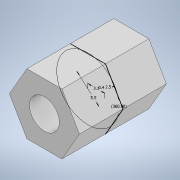
# Autodesk Inventor part: Acople_Motor_
Saved by Autodesk Inventor 2022 (Build 260153000, 153)
## iProperties
Created: 2022-03-05
Part Number: Acople_Motor_
Material: Generic
Document SubType Name: Modeling
Designer: katha
Density: 1 g/cm^3
Appearance: Default
Author: katha
Autodesk Inventor part; units mm, degrees
ref_plane "YZ Plane" through (0, 0, 0) normal (1, 0, 0) x (0, 1, 0)
ref_plane "XZ Plane" through (0, 0, 0) normal (0, 1, 0) x (-1, 0, 0)
ref_plane "XY Plane" through (0, 0, 0) normal (0, 0, 1) x (1, 0, 0)
sketch "Sketch1" plane through (0, 0, 0) normal (0, 0, 1) x (1, 0, 0)
  circle A0 centre (0, 0) radius 2.75
  line L0 (0, 0) -> (3.1, 0) construction
  line L1 (0, 0) -> (1.55, 2.6847) construction
  line L2 (0, 0) -> (-1.55, 2.6847) construction
  line L3 (0, 0) -> (-3.1, 0) construction
  line L4 (0, 0) -> (-1.55, -2.6847) construction
  line L5 (0, 0) -> (1.55, -2.6847) construction
  line L6 (-1.55, 2.6847) -> (1.55, 2.6847) construction
  line L7 (1.55, 2.6847) -> (3.1, 0) construction
  line L8 (3.1, 0) -> (1.55, -2.6847) construction
  line L9 (1.55, -2.6847) -> (-1.55, -2.6847) construction
  line L10 (-1.55, -2.6847) -> (-3.1, 0) construction
  line L11 (-3.1, 0) -> (-1.55, 2.6847) construction
  line L12 (3.5619, 0) -> (1.7809, 3.0847)
  line L13 (1.7809, 3.0847) -> (-1.7809, 3.0847)
  line L14 (-1.7809, 3.0847) -> (-3.5619, 0)
  line L15 (-3.5619, 0) -> (-1.7809, -3.0847)
  line L16 (-1.7809, -3.0847) -> (1.7809, -3.0847)
  line L17 (1.7809, -3.0847) -> (3.5619, 0)
  line L18 (3.2243, 5.5847) -> (6.4486, 0)
  line L19 (6.4486, 0) -> (3.2243, -5.5847)
  line L20 (3.2243, -5.5847) -> (-3.2243, -5.5847)
  line L21 (-3.2243, -5.5847) -> (-6.4486, 0)
  line L22 (-6.4486, 0) -> (-3.2243, 5.5847)
  line L23 (-3.2243, 5.5847) -> (3.2243, 5.5847)
  dimension "d0" = 5.5
  dimension "d2" = 3.1
  dimension "d5" = 360
  dimension "d7" = 0.4
  dimension "d8" = 2.5
  constraints: 48 end point, 9 parallel, 3 coincident, 2 horizontal, 1 centre point, 27 other
  measures "d0" diameter of A0
  measures "d2" distance of L0.start L0.end
  measures "d7" distance between parallel lines of L7 L12
  measures "d8" distance between parallel lines of L12 L18
extrude "Extrusion1" add sketch "Sketch1" along normal blind 8 contours L17 L16 L15 L14 L13 L12 | L18 L19 L20 L21 L22 L23
extrude "Extrusion2" add sketch "Sketch1" against normal blind 8 contours L18 L19 L20 L21 L22 L23
body "Solid1"
